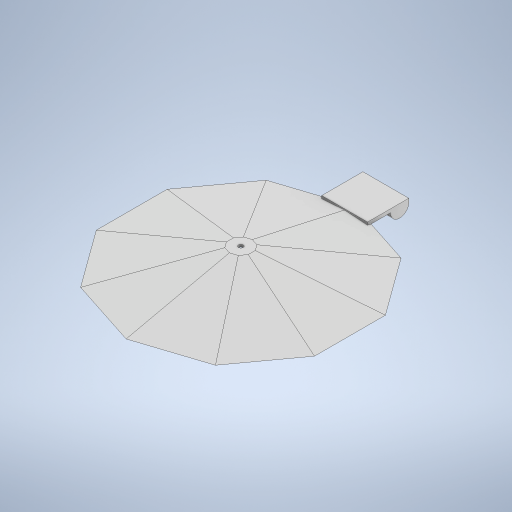
# Autodesk Inventor part: capac
Saved by Autodesk Inventor 2024 (Build 280153000, 153)
## iProperties
Created: 2024-01-15
Part Number: capac
Material: Generic
Document SubType Name: Modeling
Designer: Sorin
Density: 1 g/cm^3
Appearance: Default
Author: Sorin
Autodesk Inventor part; units mm, degrees
ref_plane "YZ Plane" through (0, 0, 0) normal (1, 0, 0) x (0, 1, 0)
ref_plane "XY Plane" through (0, 0, 0) normal (0, 0, 1) x (1, 0, 0)
sketch "Sketch1" plane through (0, 0, 0) normal (0, 1, 0) x (-1, 0, 0)
  line L0 (-29.3882, -40.4517) -> (-47.5524, -15.4522)
  line L1 (-47.5524, -15.4522) -> (-47.5533, 15.4495)
  line L2 (-47.5533, 15.4495) -> (-29.3904, 40.45)
  line L3 (-29.3904, 40.45) -> (-0.0014, 50)
  line L4 (-0.0014, 50) -> (29.3882, 40.4517)
  line L5 (29.3882, 40.4517) -> (47.5524, 15.4522)
  line L6 (47.5524, 15.4522) -> (47.5533, -15.4495)
  line L7 (47.5533, -15.4495) -> (29.3904, -40.45)
  line L8 (29.3904, -40.45) -> (0.0014, -50)
  line L9 (0.0014, -50) -> (-29.3882, -40.4517)
  point P0 (0, 0)
  point P1 (0, 0)
  dimension "d0" = 100
  dimension "d1" = 29.389
  constraints: 20 end point, 1 coincident, 21 other
  measures "d0" distance of L0.end L5.end
  measures "d1" horizontal distance of L2.end L3.end
ref_plane "Work Plane1" through (0, 10, 0) normal (0, 1, 0) x (-1, 0, 0)
sketch "Sketch2" plane through (0, 10, 0) normal (0, 1, 0) x (-1, 0, 0)
  line L0 (-2.9392, -4.0449) -> (-4.7554, -1.5447)
  line L1 (-4.7554, -1.5447) -> (-4.7552, 1.5455)
  line L2 (-4.7552, 1.5455) -> (-2.9386, 4.0453)
  line L3 (-2.9386, 4.0453) -> (0.0004, 5)
  line L4 (0.0004, 5) -> (2.9392, 4.0449)
  line L5 (2.9392, 4.0449) -> (4.7554, 1.5447)
  line L6 (4.7554, 1.5447) -> (4.7552, -1.5455)
  line L7 (4.7552, -1.5455) -> (2.9386, -4.0453)
  line L8 (2.9386, -4.0453) -> (-0.0004, -5)
  line L9 (-0.0004, -5) -> (-2.9392, -4.0449)
  point P0 (0, 0)
  point P1 (0, 0)
  dimension "d3" = 10
  dimension "d4" = 2.939
  constraints: 20 end point, 1 coincident, 21 other
  measures "d3" distance of L3.end L8.end
  measures "d4" horizontal distance of L7.end L8.end
loft "Loft1" add profiles "Sketch1", "Sketch2"
shell "Shell1" thickness 1 removed faces 1 at (-0.0005, 0, -16.6667)
sketch "Sketch4" plane through (0, 0, 0) normal (1, 0, 0) x (0, 1, 0)
  line L0 (0, -50) -> (0, -40.4517) projected
  line L1 (0, -45.2258) -> (0, -55.2258)
  line L2 (0, -45.2258) -> (1.5, -45.2258)
  line L3 (1.5, -45.2258) -> (1.5, -63.2258)
  line L4 (1.5, -63.2258) -> (0, -63.2258)
  line L5 (0, -55.2258) -> (0, -55.2258)
  arc A0 (0, -55.2258) -> (0, -63.2258) centre (0, -59.2258) ccw
  point P0 (0, 0)
  dimension "d18" = 1.5
  dimension "d21" = 4
  dimension "d22" = 18
  constraints: 10 end point, 3 perpendicular, 2 point on circle, 1 centre point, 1 collinear, 1 midpoint, 1 tangent, 1 vertical
  measures "d18" distance of L1.start L2.end
  measures "d21" radius of A0
  measures "d22" distance of L2.end L3.end
extrude "Extrusion2" add sketch "Sketch4" along normal mid plane 20
sketch "Sketch6" plane through (4.7554, 10, -1.5447) normal (0, 1, 0) x (0.8090624, 0, -0.5877228)
  line L0 (-9.5106, 3.0902) -> (-7.6942, 5.5902) construction
  line L1 (-7.6942, 5.5902) -> (-1.8373, -2.4848) construction
  line L2 (-1.8164, 5.5902) -> (0, 3.0902) construction
  line L3 (-34.1403, -38.9088) -> (-7.6942, -2.5) construction
  line L4 (-1.8164, 5.5902) -> (-7.6942, -2.5) construction
  point P0 (-4.7553, 1.5451)
  constraints: 4 end point
hole "Hole1" at (0, 10, 0) direction (0, -1, 0) diameter 2 end through all
body "Solid1"
